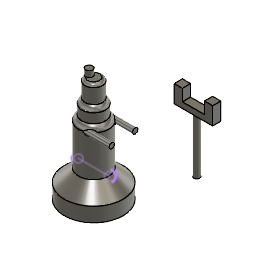
Chess- muni (Autodesk Fusion 360 design; units mm, degrees)
part number: 2026-07-02-20-24-24-744
Autodesk Fusion 360 part; units mm, degrees
sketch "Sketch1" plane through (0, 0, 0) normal (0, 0, 1) x (1, 0, 0)
  line L0 (0, 0) -> (12.7, 0)
  line L1 (0, 0) -> (0, 11.8872) construction
  line L2 (12.7, 0) -> (12.7, 5.08) construction
  line L3 (12.7, 0) -> (12.7, 6.2407)
  line L4 (0, 11.8872) -> (35.56, 11.8872) construction
  line L5 (12.7, 0) -> (12.7, 6.2407) construction
  line L6 (12.7, 6.2407) -> (6.5916, 11.8872)
  line L7 (6.5916, 11.8872) -> (6.5916, 31.8088)
  line L8 (6.5916, 31.8088) -> (5.08, 31.8088)
  line L9 (5.08, 31.8088) -> (5.08, 38.1)
  line L10 (5.08, 38.1) -> (0, 38.1)
  line L11 (0, 38.1) -> (0, 0)
  dimension "d1" = 11.8872
  constraint coincident L0.start L1.start
  constraint horizontal L0
  constraint perpendicular L0 L1
  constraint perpendicular L0 L2
  constraint perpendicular L0 L3
  constraint perpendicular L1 L4
  constraint coincident L4 L6.end
  constraint perpendicular L4 L7
  constraint perpendicular L7 L8
  constraint perpendicular L8 L9
  constraint perpendicular L9 L10
  constraint perpendicular L0 L11
  measures "d1" distance of L0.start L1.end
revolve "Revolve1" add sketch "Sketch1" angle 360 about axis through (0, 38.1, 0) along (0, -1, 0) makes body 1
sketch "Sketch2" plane through (0, 0, 0) normal (0, 0, 1) x (1, 0, 0)
sketch "Sketch3" plane through (0, 0, 0) normal (0, 0, 1) x (1, 0, 0)
  line L0 (-6.5916, 11.8872) -> (6.5916, 11.8872)
ref_plane "WorkPlane1" through (12.7, 0, 0) normal (1, 0, 0) x (0, 1, 0)
sketch "Sketch4" plane through (12.7, 0, 0) normal (1, 0, 0) x (0, 0, -1)
  line L0 (0.073, 11.8943) -> (0.073, 26.7914) construction
  line L1 (-6.35, 26.67) -> (6.604, 26.67) construction
  line L2 (6.604, 26.67) -> (-6.604, 26.67) construction
  line L3 (-6.604, 26.67) -> (6.604, 26.67) construction
  circle A0 centre (-5.08, 29.21) radius 1.27
  circle A1 centre (5.08, 29.21) radius 1.27
  dimension "d4" = 14.8971
  dimension "d5" = 2.54
  dimension "d6" = 2.54
  constraint vertical L0
  constraint perpendicular L0 L1
  constraint perpendicular L0 L2
  measures "d4" distance of L0.start L0.end
  measures "d5" diameter of A0
  measures "d6" diameter of A1
extrude "Extrude1" cut sketch "Sketch4" against normal blind 12.7 bodies 1
sketch "Sketch5" plane through (0, 0, 0) normal (1, 0, 0) x (0, 0, -1)
  circle A0 centre (25.4, 25.4) radius 1.27
  dimension "d9" = 2.54
  measures "d9" diameter of A0
sketch "Sketch12" plane through (0, 0, 0) normal (1, 0, 0) x (0, 0, -1)
sketch "Sketch9" plane through (0, 0, 0) normal (0, 0, 1) x (1, 0, 0)
  line L0 (-1.0576, -0.3775) -> (-0.7033, -0.3775)
  line L1 (-0.7033, -0.3775) -> (-0.7033, -0.5947)
  line L2 (-0.7033, -0.5947) -> (-1.0576, -0.5947)
  line L3 (-1.0576, -0.5947) -> (-1.0576, -0.3775)
  constraint horizontal L0
  constraint vertical L1
  constraint horizontal L2
  constraint vertical L3
sketch "Sketch13" plane through (0, 0, 0) normal (1, 0, 0) x (0, 0, -1)
  circle A0 centre (-38.1, 12.7) radius 1.143
  dimension "d26" = 2.286
  measures "d26" diameter of A0
extrude "Extrude9" add sketch "Sketch13" along normal blind 12.7 separate body makes body 2
sketch "Sketch14" plane through (12.7, 0, 0) normal (1, 0, 0) x (0, 0, -1)
  circle A0 centre (-38.1, 12.7) radius 1.143
  line L0 (-38.862, 12.7) -> (-37.338, 12.7)
  line L1 (-37.338, 12.7) -> (-37.338, 11.938)
  line L2 (-37.338, 11.938) -> (-38.862, 11.938)
  line L3 (-38.862, 11.938) -> (-38.862, 12.7)
  constraint horizontal L0
  constraint vertical L1
  constraint horizontal L2
  constraint vertical L3
extrude "Extrude10" add sketch "Sketch14" along normal blind 1.27 contours L0 L1 L2 L3 bodies 2
sketch "Sketch15" plane through (0, 12.7, 0) normal (0, 1, 0) x (-1, 0, 0)
  line L0 (-12.7, 37.338) -> (-12.7, 38.862)
  line L1 (-12.7, 38.862) -> (-13.97, 38.862)
  line L2 (-13.97, 38.862) -> (-13.97, 37.338)
  line L3 (-13.97, 37.338) -> (-12.7, 37.338)
  line L4 (-13.97, 38.862) -> (-13.3865, 38.862)
  line L5 (-13.3865, 38.862) -> (-13.3865, 37.338)
  line L6 (-13.3865, 37.338) -> (-13.97, 37.338)
  line L7 (-13.97, 37.338) -> (-13.97, 38.862)
  constraint horizontal L4
  constraint vertical L5
  constraint horizontal L6
  constraint vertical L7
  constraint coincident L3 L5.end
  constraint coincident L1.end L2.start
extrude "Extrude11" add sketch "Sketch15" along normal blind 0.254 contours L1 L2 L3 L4 L5 L6 L7 bodies 2
copy_body "CopyPasteBodies1" bodies 2 makes body 3
move_body "Move5" bodies 3 to x (1, 0, 0) y (0, 1, 0) z (0, 0, 1) at (0, 0, 12.7)
move_body "Move6" bodies 2 to x (1, 0, 0) y (0, 1, 0) z (0, 0, 1) at (0.254, 15.5683, -35.2714)
move_body "Move7" bodies 2 to x (1, 0, 0) y (0, 1, 0) z (0, 0, 1) at (0, 0.762, 2.286)
move_body "Move8" bodies 3 to x (1, 0, 0) y (0, 1, 0) z (0, 0, 1) at (0, 16.51, -56.134)
delete_face "DeleteFace2" 6 faces at (13.97, 28.7867, -5.08) (13.3522, 28.702, -4.572) (13.7755, 29.464, -5.588) (12.9288, 29.21, -5.08) (13.3522, 28.702, -6.096) (13.1233, 28.448, -5.588) on bodies 3
sketch "Sketch16" plane through (0, 0, 0) normal (1, 0, 0) x (0, 0, -1)
sketch "Sketch17" plane through (0, 0, 0) normal (1, 0, 0) x (0, 0, -1)
  circle A0 centre (25.4, 12.7) radius 1.27
  dimension "d33" = 2.54
  measures "d33" diameter of A0
extrude "Extrude12" add sketch "Sketch17" along normal blind 50.8 separate body makes body 4
sketch "Sketch18" plane through (0, 0, 0) normal (0, 0, 1) x (1, 0, 0)
extrude "Extrude13" add 1 faces at (12.7, 29.4691, -5.7829) along direction (1, 0, 0) blind 1.27 on bodies 3 bodies 3
extrude "Extrude14" cut 1 faces at (13.97, 29.4691, -5.7829) along direction (-1, 0, 0) blind 1.27 on bodies 3 bodies 3
extrude "Extrude15" cut 1 faces at (50.8, 12.8248, -24.9955) along direction (-1, 0, 0) blind 25.4 on bodies 4 bodies 4
move_body "Move9" bodies 4 to x (0, 1, 0) y (-1, 0, 0) z (0, 0, 1) at (24.13, 16.51, 20.066)
move_body "Move10" bodies 4 to x (1, 0, 0) y (0, 1, 0) z (0, 0, 1) at (2.54, 0, 0)
sketch "Sketch19" plane through (0, 41.91, 0) normal (0, 1, 0) x (-1, 0, 0)
  circle A0 centre (-13.97, -5.334) radius 1.27
  line L0 (-15.1612, -1.524) -> (-12.7788, -1.524)
  line L1 (-12.7788, -1.524) -> (-12.7788, -9.144)
  line L2 (-12.7788, -9.144) -> (-15.1612, -9.144)
  line L3 (-15.1612, -9.144) -> (-15.1612, -1.524)
  line L4 (-15.1612, -1.524) -> (-12.7788, -9.144) construction
  line L5 (-12.7788, -1.524) -> (-15.1612, -9.144) construction
  point P0 (-13.97, -5.334)
  dimension "d42" = 7.62
  constraint horizontal L0
  constraint perpendicular L0 L1
  constraint parallel L0 L2
  constraint parallel L1 L3
  constraint coincident L4 P0
  constraint coincident L5 P0
  constraint coincident P0 A0.centre
  measures "d42" distance of L0.end L1.end
sketch "Sketch20" plane through (0, 42.164, 0) normal (0, 1, 0) x (-1, 0, 0)
  arc A0 (-12.7788, -4.8936) -> (-15.1612, -4.8936) centre (-13.97, -5.334) ccw
  line L0 (-12.7788, -4.8936) -> (-12.7788, -1.524)
  line L1 (-12.7788, -1.524) -> (-15.1612, -1.524)
  line L2 (-15.1612, -1.524) -> (-15.1612, -4.8936)
  line L3 (-12.7788, -1.524) -> (-15.1612, -1.524)
  line L4 (-15.1612, -1.524) -> (-15.1612, -2.794)
  line L5 (-15.1612, -2.794) -> (-12.7788, -2.794)
  line L6 (-12.7788, -2.794) -> (-12.7788, -1.524)
  line L7 (-15.24, -9.144) -> (-12.7, -9.144)
  line L8 (-12.7, -9.144) -> (-12.7, -8.128)
  line L9 (-12.7, -8.128) -> (-15.24, -8.128)
  line L10 (-15.24, -8.128) -> (-15.24, -9.144)
  dimension "d45" = 1.27
  constraint horizontal L3
  constraint vertical L4
  constraint horizontal L5
  constraint vertical L6
  constraint coincident L0.end L1.start
  constraint horizontal L7
  constraint vertical L8
  constraint horizontal L9
  constraint vertical L10
  measures "d45" distance of L0.end L5.end
sketch "Sketch21" plane through (0, 38.1, 0) normal (0, 1, 0) x (-1, 0, 0)
  circle A0 centre (0, 0) radius 5.08
  circle A1 centre (0, 0) radius 3.81
  dimension "d48" = 7.62
  constraint coincident A0.centre A1.centre
  measures "d48" diameter of A1
extrude "Extrude18" add sketch "Sketch21" along normal blind 7.62 contours A1 bodies 1
sketch "Sketch22" plane through (0, 45.72, 0) normal (0, 1, 0) x (-1, 0, 0)
  circle A0 centre (0, 0) radius 3.81
  circle A1 centre (1.9106, 0.0403) radius 1.5484
extrude "Extrude19" add sketch "Sketch22" along normal blind 2.54 contours A1 bodies 1
fillet "Fillet1" radius 2.54 1 edges at (-6.1455, 31.8088, -2.3836) on bodies 1
fillet "Fillet2" radius 2.54 1 edges at (-4.7362, 38.1, -1.837) on bodies 1
fillet "Fillet3" radius 1.27 1 edges at (3.5522, 45.72, -1.3778) on bodies 1
ref_plane "WorkPlane3" through (12.7, 0, 0) normal (1, 0, 0) x (0, 1, 0)
sketch "Sketch23" plane through (12.7, 0, 0) normal (1, 0, 0) x (0, 0, -1)
  line L0 (-10.16, -2.54) -> (9.5495, -2.54)
  line L1 (9.5495, -2.54) -> (9.5495, -5.08)
  line L2 (9.5495, -5.08) -> (-10.16, -5.08)
  line L3 (-10.16, -5.08) -> (-10.16, -2.54)
  dimension "d60" = 2.54
  constraint horizontal L0
  constraint vertical L1
  constraint horizontal L2
  constraint vertical L3
  measures "d60" distance of L0.start L2.end
sketch "Sketch24" plane through (0, 0, 0) normal (0, 0, 1) x (1, 0, 0)
move_body "Move14" bodies 4 to x (1, 0, 0) y (0, 1, 0) z (0, 0, 1) at (0, 0, -25.4)
sketch "Sketch28" plane through (0, 0, 0) normal (0, 1, 0) x (1, 0, 0)
  line L0 (5.8597, 32.5761) -> (22.545, 32.5761)
  line L1 (22.545, 32.5761) -> (22.545, 29.0007)
  line L2 (22.545, 29.0007) -> (5.8597, 29.0007)
  line L3 (5.8597, 29.0007) -> (5.8597, 32.5761)
  line L4 (5.8597, 32.5761) -> (22.545, 29.0007) construction
  line L5 (22.545, 32.5761) -> (5.8597, 29.0007) construction
  point P0 (14.2024, 30.7884)
  constraint horizontal L0
  constraint perpendicular L0 L1
  constraint parallel L0 L2
  constraint parallel L1 L3
  constraint coincident L4 P0
  constraint coincident L5 P0
extrude "Extrude21" add sketch "Sketch28" along normal blind 2.54 separate body makes body 5
sketch "Sketch29" plane through (0, 2.54, 0) normal (0, 1, 0) x (-1, 0, 0)
  line L0 (-5.8597, -29.0007) -> (-22.545, -29.0007)
  line L1 (-22.545, -29.0007) -> (-22.545, -32.5761)
  line L2 (-22.545, -32.5761) -> (-5.8597, -32.5761)
  line L3 (-5.8597, -32.5761) -> (-5.8597, -29.0007)
  line L4 (-22.545, -29.0007) -> (-18.9694, -29.0007)
  line L5 (-18.9694, -29.0007) -> (-18.9694, -32.5761)
  line L6 (-18.9694, -32.5761) -> (-22.545, -32.5761)
  line L7 (-22.545, -32.5761) -> (-22.545, -29.0007)
  line L8 (-5.8597, -29.0007) -> (-9.4411, -29.0007)
  line L9 (-9.4411, -29.0007) -> (-9.4411, -32.5821)
  line L10 (-9.4411, -32.5821) -> (-5.8597, -32.5821)
  line L11 (-5.8597, -32.5821) -> (-5.8597, -29.0007)
  dimension "d66" = 3.5814
  dimension "d67" = 3.5814
  constraint horizontal L4
  constraint vertical L5
  constraint horizontal L6
  constraint vertical L7
  constraint coincident L2 L5.end
  constraint coincident L0.end L1.start
  constraint horizontal L8
  constraint vertical L9
  constraint horizontal L10
  constraint vertical L11
  constraint coincident L0.start L3.end
  measures "d66" distance of L0.start L8.end
  measures "d67" distance of L0.start L10.end
extrude "Extrude22" add sketch "Sketch29" along normal blind 5.08 contours L0 L2 L3 L8 L9 L11 | L0 L1 L2 L4 L5 L6 L7 bodies 5
move_body "Move15" bodies 5 to x (1, 0, 0) y (0, 1, 0) z (0, 0, 1) at (0, 40.64, 0)
combine "Combine3" operation add target body 5 tool bodies 4
delete_face "DeleteFace3" 4 faces at (14.224, 28.9457, 5.3686) (14.0295, 29.2843, 4.8606) (13.6062, 28.5223, 5.8766) (13.1828, 29.0303, 5.3686) on bodies 2
move_body "Move16" bodies 5 to x (1, 0, 0) y (0, 1, 0) z (0, 0, 1) at (0, -16.51, 0)
move_body "Move11" [suppressed]
move_body "Move12" [suppressed]
move_body "Move13" [suppressed]
sketch "Sketch25" plane through (0, 0, 0) normal (0, 1, 0) x (1, 0, 0)
  circle A0 centre (0, 0) radius 3.81
  dimension "d63" = 7.62
  constraint coincident A0.centre origin
  measures "d63" diameter of A0
sketch "Sketch26" plane through (0, 0, 0) normal (0, 1, 0) x (1, 0, 0)
sketch "Sketch27" plane through (0, 0, 0) normal (1, 0, 0) x (0, 0, -1)
equation "d4 = ( 0.782 * 0.75 ) * 1 in"
named bodies: "19"
